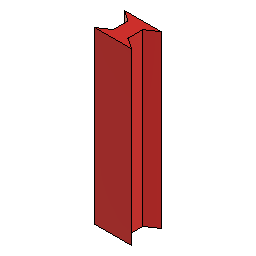
Prindere zid (Autodesk Fusion 360 design; units mm, degrees)
part number: 2026-06-02-22-23-02-650
Autodesk Fusion 360 part; units mm, degrees
sketch "Sketch1" plane through (0, 0, 0) normal (0, 0, 1) x (1, 0, 0)
  line L0 (125, 0) -> (125, 1)
  line L1 (127, 0) -> (127, 1)
  line L2 (125, 0) -> (127, 0)
  line L3 (126, 0) -> (126, 2) construction
  line L4 (123.5, 2) -> (128.5, 2)
  line L5 (123.5, 2) -> (125, 1)
  line L6 (127, 1) -> (128.5, 2)
  line L7 (125, 0) -> (125, -1)
  line L8 (123.5, -2) -> (125, -1)
  line L9 (123.5, -2) -> (128.5, -2)
  line L10 (127, -1) -> (128.5, -2)
  line L11 (127, 0) -> (127, -1)
  line L12 (125, 0) -> (127, 0)
  dimension "d759" = 1
  dimension "d760" = 1
  dimension "d761" = 2
  dimension "d763" = 2
  dimension "d764" = 5
  constraint vertical L0
  constraint vertical L1
  constraint perpendicular L1 L2
  constraint midpoint L2 L3.start
  constraint perpendicular L2 L3
  constraint midpoint L3.end L4
  constraint perpendicular L3 L4
  constraint symmetric L0.start L2 L7.start
  constraint symmetric L0.end L2 L7.end
  constraint symmetric L1.start L2 L11.start
  constraint symmetric L1.end L2 L10.start
  constraint symmetric L2 L4.start L8.start
  constraint symmetric L2 L4.end L9.end
  measures "d759" distance of L0.start L0.end
  measures "d760" distance of L1.start L1.end
  measures "d761" distance of L0 L1
  measures "d763" distance of L3.start L3.end
  measures "d764" distance of L4.start L4.end
extrude "Extrude1" add sketch "Sketch1" along normal blind 23
named bodies: "Poarta Dreapta Sus"
